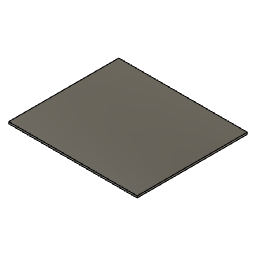
USB_Plastic_Plate (Autodesk Fusion 360 design; units mm, degrees)
Autodesk Fusion 360 part; units mm, degrees
sketch "Skizze1" plane through (0, 0, 0) normal (0, 0, 1) x (1, 0, 0)
  line L0 (7, -6) -> (-7, -6)
  line L1 (-7, -6) -> (-7, 6)
  line L2 (-7, 6) -> (7, 6)
  line L3 (7, 6) -> (7, -6)
  line L4 (7, -6) -> (-7, 6) construction
  line L5 (-7, -6) -> (7, 6) construction
  dimension "d1" = 14
  dimension "d2" = 12
  constraint horizontal L0
  constraint perpendicular L0 L1
  constraint parallel L0 L2
  constraint parallel L1 L3
  constraint coincident L4 origin
  constraint coincident L5 origin
  measures "d1" distance of L1.end L2.end
  measures "d2" distance of L0.end L1.end
extrude "Extrusion1" add sketch "Skizze1" along normal blind 0.2
